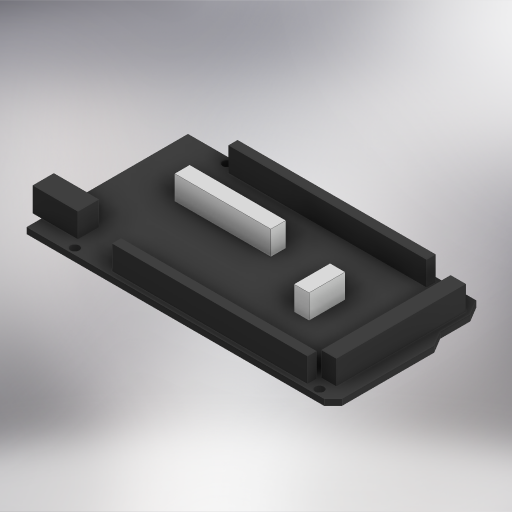
# Autodesk Inventor part: Wemos Mega
Saved by Autodesk Inventor 2024 (Build 280153000, 153)
## iProperties
Created: 2023-11-01
Part Number: Wemos Mega
Material: Genérico
Document SubType Name: Modeling
Designer: juesr
Density: 1 g/cm^3
Appearance: Valor por defecto
Author: juesr
Autodesk Inventor part; units mm, degrees
ref_plane "YZ Plane" through (0, 0, 0) normal (1, 0, 0) x (0, 1, 0)
ref_plane "XZ Plane" through (0, 0, 0) normal (0, 1, 0) x (-1, 0, 0)
ref_plane "XY Plane" through (0, 0, 0) normal (0, 0, 1) x (1, 0, 0)
sketch "Boceto1" plane through (0, 0, 0) normal (0, 1, 0) x (-1, 0, 0)
  line L0 (70.0475, 27.7623) -> (-31.8125, 27.7623)
  line L1 (-31.8125, 27.7623) -> (-31.8125, -25.8477)
  line L2 (-31.8125, -25.8477) -> (70.0475, -25.8477)
  line L3 (70.0475, -25.8477) -> (70.0475, 27.7623)
  point P0 (0, 0)
  dimension "d0" = 53.61
  dimension "d1" = 101.86
  constraints: 8 end point, 2 parallel, 1 horizontal, 1 perpendicular
  measures "d0" distance between parallel lines of L2 L0
  measures "d1" distance between parallel lines of L1 L3
extrude "Extrusión1" add sketch "Boceto1" along normal blind 2
sketch "Boceto6" plane through (0, 0, 0) normal (0, -1, 0) x (1, 0, 0)
  line L0 (-50.0475, 27.7623) -> (23.8125, 27.7623) projected
  line L1 (28.8125, 27.7623) -> (31.8125, 24.7623)
  line L2 (31.8125, 27.7623) -> (31.8125, -25.8477) projected
  line L3 (-70.0475, 27.7623) -> (31.8125, 27.7623) projected
  line L4 (28.8125, 27.7623) -> (31.8125, 27.7623)
  line L5 (31.8125, 27.7623) -> (31.8125, 24.7623)
  circle A0 centre (25.3125, 25.7623) radius 1.5
  line L6 (31.8125, 17.7623) -> (31.8125, -25.8477) projected
  line L7 (31.8125, -15.8477) -> (25.8125, -25.8477)
  line L8 (31.8125, -25.8477) -> (23.8125, -25.8477) projected
  line L9 (31.8125, -25.8477) -> (28.8125, -25.8477)
  line L10 (28.8125, -25.8477) -> (28.8125, 5.0493)
  line L11 (28.8125, -10.8477) -> (31.8125, -5.8477)
  line L12 (31.8125, -5.8477) -> (31.8125, -25.8477)
  line L13 (25.8125, -25.8477) -> (31.8125, -25.8477)
  circle A1 centre (16.8125, -23.8477) radius 1.5
  line L14 (31.8125, -25.8477) -> (-70.0475, -25.8477) projected
  circle A2 centre (-56.0475, 25.7623) radius 1.5
  line L15 (-70.0475, 27.7623) -> (31.8125, 27.7623) projected
  line L16 (-70.0475, -25.8477) -> (-70.0475, 27.7623) projected
  circle A3 centre (-55.0475, -23.8477) radius 1.5
  point P0 (0, 0)
  point P1 (28.8125, -20.8477)
  point P2 (28.8125, -20.8477)
  dimension "d39" = 3
  dimension "d40" = 3
  dimension "d41" = 3
  dimension "d42" = 6.5
  dimension "d43" = 2
  dimension "d44" = 6
  dimension "d45" = 10
  dimension "d46" = 3
  dimension "d47" = 10
  dimension "d48" = 10
  dimension "d49" = 3
  dimension "d50" = 2
  dimension "d51" = 15
  dimension "d52" = 3
  dimension "d53" = 2
  dimension "d54" = 14
  dimension "d55" = 3
  dimension "d56" = 2
  dimension "d57" = 15
  constraints: 18 end point, 7 point on line, 4 centre point, 4 collinear, 1 midpoint, 1 perpendicular
  measures "d39" distance of L2.start L1.start
  measures "d40" distance of L2.start L1.end
  measures "d41" diameter of A0
  measures "d42" distance from line of L2 A0.centre
  measures "d43" vertical distance of L0.end A0.centre
  measures "d44" distance of L7.end L2.end
  measures "d45" distance of L2.end L7.start
  measures "d46" distance of L2.end L9.end
  measures "d47" distance of L11.start point (28.813, -20.848)
  measures "d48" distance of L7.start L11.end
  measures "d49" diameter of A1
  measures "d50" distance from line of L14 A1.centre
  measures "d51" distance from line of L6 A1.centre
  measures "d52" diameter of A2
  measures "d53" distance from line of L15 A2.centre
  measures "d54" distance from line of L16 A2.centre
  measures "d55" diameter of A3
  measures "d56" distance from line of L14 A3.centre
  measures "d57" distance from line of L16 A3.centre
extrude "Extrusión7" cut sketch "Boceto6" against normal blind 3 contours L3 L2 L1 | L7 L10 L8 | L2 L7 L10 L11 | L7 L2 L8 L10 | A0 | A1 | A2 | A3
sketch "Boceto5" plane through (0, 2, 0) normal (0, 1, 0) x (1, 0, 0)
  line L0 (-73.0475, -22.7623) -> (-58.0475, -22.7623)
  line L1 (-58.0475, -22.7623) -> (-58.0475, -15.7623)
  line L2 (-58.0475, -15.7623) -> (-73.0475, -15.7623)
  line L3 (-73.0475, -15.7623) -> (-73.0475, -22.7623)
  line L4 (-70.0475, -27.7623) -> (31.8125, -27.7623) projected
  line L5 (-70.0475, 25.8477) -> (-70.0475, -27.7623) projected
  point P0 (0, 0)
  point P1 (-50.0475, -27.7623)
  point P2 (-65.5475, -22.7623)
  dimension "d33" = 5
  dimension "d34" = 7
  dimension "d35" = 3
  dimension "d36" = 15
  constraints: 8 end point, 2 parallel, 1 horizontal, 1 midpoint, 1 perpendicular
  measures "d33" distance between parallel lines of L4 L0
  measures "d34" distance from line of L2 point (-65.547, -22.762)
  measures "d35" distance between parallel lines of L3 L5
  measures "d36" distance between parallel lines of L1 L3
extrude "Extrusión6" add sketch "Boceto5" along normal blind 8
sketch "Boceto4" plane through (0, 2, 0) normal (0, 1, 0) x (1, 0, 0)
  line L0 (-52.9032, 4.2581) -> (-20.9032, 4.2581)
  line L1 (-20.9032, 4.2581) -> (-20.9032, 9.2581)
  line L2 (-20.9032, 9.2581) -> (-52.9032, 9.2581)
  line L3 (-52.9032, 9.2581) -> (-52.9032, 4.2581)
  line L4 (-1.1875, -7.7419) -> (3.8125, -7.7419)
  line L5 (3.8125, -7.7419) -> (3.8125, 4.2581)
  line L6 (3.8125, 4.2581) -> (-1.1875, 4.2581)
  line L7 (-1.1875, 4.2581) -> (-1.1875, -7.7419)
  line L8 (23.8125, 25.8477) -> (23.8125, -17.7623) projected
  point P0 (0, 0)
  point P1 (-36.9032, 9.2581)
  point P2 (-36.9032, 4.2581)
  point P3 (1.3125, 4.2581)
  point P4 (1.3125, -7.7419)
  point P5 (-1.1875, -1.7419)
  point P6 (3.8125, -1.7419)
  point P7 (-20.9032, 6.7581)
  point P8 (-52.9032, 6.7581)
  dimension "d19" = 5
  dimension "d20" = 12
  dimension "d21" = 5
  dimension "d22" = 32
  dimension "d23" = 20
  constraints: 16 end point, 8 midpoint, 4 parallel, 2 horizontal, 2 perpendicular, 1 point on line
  measures "d19" distance of point (-36.903, 9.258) point (-36.903, 4.258)
  measures "d20" distance of point (1.313, 4.258) point (1.313, -7.742)
  measures "d21" distance of point (-1.187, -1.742) point (3.813, -1.742)
  measures "d22" distance of point (-20.903, 6.758) point (-52.903, 6.758)
  measures "d23" distance between parallel lines of L8 L5
extrude "Extrusión4" add sketch "Boceto4" along normal blind 8
sketch "Boceto7" plane through (0, 2, 0) normal (0, 1, 0) x (1, 0, 0)
  line L0 (27.3125, 20.8477) -> (22.3125, 20.8477)
  line L1 (22.3125, 20.8477) -> (22.3125, -22.1523)
  line L2 (22.3125, -22.1523) -> (27.3125, -22.1523)
  line L3 (27.3125, -22.1523) -> (27.3125, 20.8477)
  line L4 (28.8125, 10.8477) -> (28.8125, 20.8477) projected
  line L5 (25.8125, 25.8477) -> (-70.0475, 25.8477) projected
  line L6 (21.8125, -23.2623) -> (-43.1875, -23.2623)
  line L7 (-43.1875, -23.2623) -> (-43.1875, -26.2623)
  line L8 (-43.1875, -26.2623) -> (21.8125, -26.2623)
  line L9 (21.8125, -26.2623) -> (21.8125, -23.2623)
  line L10 (-70.0475, -27.7623) -> (28.8125, -27.7623) projected
  line L11 (31.8125, -24.7623) -> (31.8125, 5.8477) projected
  line L12 (13.8125, 24.3477) -> (-52.0475, 24.3477)
  line L13 (-52.0475, 24.3477) -> (-52.0475, 21.3477)
  line L14 (-52.0475, 21.3477) -> (13.8125, 21.3477)
  line L15 (13.8125, 21.3477) -> (13.8125, 24.3477)
  line L16 (-70.0475, 25.8477) -> (-70.0475, -15.7623) projected
  point P0 (0, 0)
  point P1 (24.8125, 20.8477)
  point P2 (21.8125, -24.7623)
  point P3 (-43.1875, -24.7623)
  point P4 (13.8125, 22.8477)
  point P5 (-52.0475, 22.8477)
  dimension "d60" = 1.5
  dimension "d61" = 5
  dimension "d62" = 5
  dimension "d63" = 43
  dimension "d64" = 1.5
  dimension "d65" = 3
  dimension "d66" = 10
  dimension "d67" = 65
  dimension "d68" = 1.5
  dimension "d69" = 3
  dimension "d70" = 15
  dimension "d71" = 18
  constraints: 24 end point, 6 parallel, 5 midpoint, 3 horizontal, 3 perpendicular
  measures "d60" distance between parallel lines of L4 L3
  measures "d61" distance between parallel lines of L3 L1
  measures "d62" distance from line of L5 point (24.813, 20.848)
  measures "d63" distance between parallel lines of L2 L0
  measures "d64" distance between parallel lines of L10 L8
  measures "d65" distance between parallel lines of L8 L6
  measures "d66" distance from line of L11 point (21.813, -24.762)
  measures "d67" distance from line of point (-43.187, -24.762) L9
  measures "d68" distance between parallel lines of L5 L12
  measures "d69" distance between parallel lines of L12 L14
  measures "d70" distance from line of L4 point (13.813, 22.848)
  measures "d71" distance from line of L16 point (-52.047, 22.848)
extrude "Extrusión8" add sketch "Boceto7" along normal blind 8
